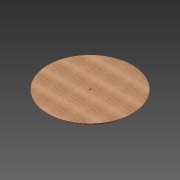
# Autodesk Inventor part: bottom
Saved by Autodesk Inventor 2013 (Build 170138000, 138)
## iProperties
Created: 2013-04-07
Part Number: bottom
Material: Wood (Birch)
Document SubType Name: Modeling
Designer: Chris
Density: 1 g/cm^3
Mass: 22228.7 g
Surface Area: 24094.6 cm^2
Volume: 22228.7 cm^3
Author: Chris
Autodesk Inventor part; units mm, degrees
ref_plane "YZ Plane" through (0, 0, 0) normal (1, 0, 0) x (0, 1, 0)
ref_plane "XZ Plane" through (0, 0, 0) normal (0, 1, 0) x (-1, 0, 0)
ref_plane "XY Plane" through (0, 0, 0) normal (0, 0, 1) x (1, 0, 0)
sketch "Sketch1" plane through (0, 0, 0) normal (0, 1, 0) x (-1, 0, 0)
  circle A0 centre (0, 0) radius 609.6
  circle A1 centre (0, 0) radius 12.7
  circle A2 centre (0, 596.9) radius 2.6035
  line L0 (0, 12.7) -> (0, 594.2965)
  circle A3 centre (-596.9, 0) radius 2.6035
  circle A4 centre (0, -596.9) radius 2.6035
  circle A5 centre (596.9, 0) radius 2.6035
  point P0 (-594.2965, 0)
  point P1 (0, -594.2965)
  point P2 (594.2965, 0)
  dimension "d5" = 25.4
  dimension "d6" = 5.207
  dimension "d0" = 1219.2
  dimension "d7" = 596.9
  dimension "d10" = 360
  constraints: 4 vertical alignment, 2 coincident, 2 end point, 2 horizontal alignment, 2 vertical, 1 centre point, 23 other
  measures "d0" diameter of A0
  measures "d7" distance of A0.centre point (0, 596.9)
extrude "Extrusion1" add sketch "Sketch1" along normal blind 19.05
body "Solid1"
